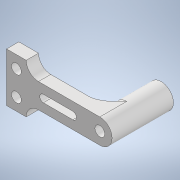
# Autodesk Inventor part: arm_holder_2
Saved by Autodesk Inventor 2020 (Build 240168000, 168)
## iProperties
Created: 2020-01-20
Part Number: arm_holder_2
Material: Generic
Document SubType Name: Modeling
Designer: psrobotics
Density: 1 g/cm^3
Appearance: Default
Author: psrobotics
Autodesk Inventor part; units mm, degrees
ref_plane "YZ Plane" through (0, 0, 0) normal (1, 0, 0) x (0, 1, 0)
ref_plane "XZ Plane" through (0, 0, 0) normal (0, 1, 0) x (-1, 0, 0)
ref_plane "XY Plane" through (0, 0, 0) normal (0, 0, 1) x (1, 0, 0)
sketch "Sketch1" plane through (0, 0, 0) normal (0, 0, 1) x (1, 0, 0)
  circle A0 centre (13.5, 6) radius 2 projected
  circle A1 centre (13.5, 6) radius 5
  point P0 (0, 0)
  dimension "d0" = 10
  constraints: 1 centre point, 1 coincident
  measures "d0" diameter of A1
extrude "Extrusion1" add sketch "Sketch1" along normal blind 20
sketch "Sketch2" plane through (13.5, 6, 20) normal (0, 0, 1) x (1, 0, 0)
  circle A0 centre (0, 0) radius 5 projected
  circle A1 centre (0, 0) radius 2 projected
  circle A2 centre (0, 0) radius 5 projected
  line L0 (0, 5) -> (-30, 5)
  line L1 (-30, 5) -> (-30, -5)
  line L2 (-30, -5) -> (0, -5)
  line L3 (0, -5) -> (0, 5)
  line L4 (0, 0) -> (0, 5)
  point P0 (-13.5, -6)
  point P1 (0, -5)
  dimension "d3" = 30
  dimension "d4" = 10
  constraints: 10 end point, 2 parallel, 1 horizontal, 1 perpendicular, 1 vertical, 1 vertical alignment, 1 other
  measures "d3" distance of L2.end L1.end
  measures "d4" distance of L1.end L0.end
extrude "Extrusion2" add sketch "Sketch2" along normal blind 5
sketch "Sketch3" plane through (13.5, 6, 25) normal (0, 0, 1) x (1, 0, 0)
  circle A0 centre (0, 0) radius 2 projected
  point P0 (-13.5, -6)
extrude "Extrusion3" cut sketch "Sketch3" against normal blind 5
fillet "Fillet1" radius 6 1 edges at (8.5, 6, 20)
sketch "Sketch4" plane through (13.5, 6, 25) normal (0, 0, 1) x (1, 0, 0)
  circle A0 centre (0, 0) radius 2 projected
  line L0 (-30, 5) -> (-30, -5) projected
  line L1 (-30, -5) -> (0, -5) projected
  arc A1 (0, -5) -> (0, 5) centre (0, 0) ccw projected
  line L2 (0, 5) -> (-30, 5) projected
  line L3 (-30, 0) -> (-34, 0)
  line L4 (-38, 10) -> (-30, 10)
  line L5 (-30, 10) -> (-30, -10)
  line L6 (-30, -10) -> (-38, -10)
  line L7 (-38, -10) -> (-38, 10)
  line L8 (-38, 10) -> (-30, -10) construction
  line L9 (-30, 10) -> (-38, -10) construction
  point P0 (-13.5, -6)
  dimension "d10" = 4
  dimension "d11" = 8
  dimension "d12" = 20
  constraints: 14 end point, 3 midpoint, 3 parallel, 1 horizontal, 1 perpendicular
  measures "d10" distance of L3.start L3.end
  measures "d11" distance of L4.start L4.end
  measures "d12" distance of L4.end L5.end
extrude "Extrusion4" add sketch "Sketch4" against normal blind 5 contours L0 L5 L6 L7 L4
sketch "Sketch5" plane through (13.5, 6, 25) normal (0, 0, 1) x (1, 0, 0)
  circle A0 centre (0, 0) radius 2 projected
  line L0 (-30, -5) -> (0, -5) projected
  arc A1 (0, -5) -> (0, 5) centre (0, 0) ccw projected
  line L1 (0, 5) -> (-30, 5) projected
  line L2 (-30, 5) -> (-30, 10) projected
  line L3 (-30, 10) -> (-38, 10) projected
  line L4 (-38, 10) -> (-38, -10) projected
  line L5 (-38, -10) -> (-30, -10) projected
  line L6 (-30, -10) -> (-30, -5) projected
  line L7 (-30, 10) -> (-38, 10) projected
  line L8 (-34, 10) -> (-34, 5)
  line L9 (-38, -10) -> (-30, -10) projected
  line L10 (-34, -10) -> (-34, -5)
  circle A2 centre (-34, 5) radius 2
  circle A3 centre (-34, -5) radius 2
  point P0 (-13.5, -6)
  dimension "d15" = 5
  dimension "d16" = 5
  dimension "d17" = 4
  dimension "d18" = 4
  constraints: 4 end point, 2 centre point, 2 coincident, 2 midpoint, 2 vertical
  measures "d15" distance of L8.start L8.end
  measures "d16" distance of L10.start L10.end
  measures "d17" diameter of A2
  measures "d18" diameter of A3
extrude "Extrusion5" cut sketch "Sketch5" against normal blind 5 contours A2 | A3
fillet "Fillet2" radius 5 2 edges at (-16.5, 1, 22.5) (-16.5, 11, 22.5)
sketch "Sketch6" plane through (13.5, 6, 25) normal (0, 0, 1) x (1, 0, 0)
  circle A0 centre (-34, -5) radius 2 projected
  circle A1 centre (-34, 5) radius 2 projected
  circle A2 centre (0, 0) radius 2 projected
  line L0 (-25, -5) -> (0, -5) projected
  arc A3 (0, -5) -> (0, 5) centre (0, 0) ccw projected
  line L1 (0, 5) -> (-25, 5) projected
  arc A4 (-30, 10) -> (-25, 5) centre (-25, 10) ccw projected
  line L2 (-30, 10) -> (-38, 10) projected
  line L3 (-38, 10) -> (-38, -10) projected
  line L4 (-38, -10) -> (-30, -10) projected
  arc A5 (-25, -5) -> (-30, -10) centre (-25, -10) ccw projected
  line L5 (0, 0) -> (-17, 0)
  line L6 (-23, 0) -> (-11, 0) construction
  line L7 (-23, -1.5) -> (-11, -1.5)
  line L8 (-11, 1.5) -> (-23, 1.5)
  arc A6 (-23, 1.5) -> (-23, -1.5) centre (-23, 0) ccw
  arc A7 (-11, -1.5) -> (-11, 1.5) centre (-11, 0) ccw
  point P0 (-13.5, -6)
  dimension "d22" = 17
  dimension "d23" = 6
  dimension "d24" = 3
  constraints: 10 end point, 4 point on circle, 4 tangent, 2 centre point, 1 horizontal, 1 midpoint, 1 parallel, 1 point on line
  measures "d22" distance of L5.start L5.end
  measures "d23" distance of L5.end L6.end
  measures "d24" diameter of A7
extrude "Extrusion6" cut sketch "Sketch6" against normal blind 8 contours A6 L8 A7 L7
body "Solid1"
